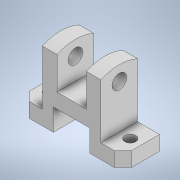
# Autodesk Inventor part: AnchorBase
Saved by Autodesk Inventor 2022.2 (Build 262287030, 287C)
## iProperties
Created: 2023-03-24
Part Number: AnchorBase
Material: Generic
Document SubType Name: Modeling
Designer: jak27277
Mass: 66.295 g
Surface Area: 179.577 cm^2
Volume: 66.295 cm^3
Density: 1 g/cm^3
Appearance: Default
Author: jak27277
Autodesk Inventor part; units mm, degrees
ref_plane "YZ Plane" through (0, 0, 0) normal (1, 0, 0) x (0, 1, 0)
ref_plane "XZ Plane" through (0, 0, 0) normal (0, 1, 0) x (-1, 0, 0)
ref_plane "XY Plane" through (0, 0, 0) normal (0, 0, 1) x (1, 0, 0)
sketch "Sketch2" plane through (0, 0, 0) normal (1, 0, 0) x (0, 1, 0)
  line L0 (-23.6676, 15.875) -> (23.6676, 15.875)
  line L1 (23.6676, 15.875) -> (23.6676, -15.875) construction
  line L2 (23.6676, -15.875) -> (-23.6676, -15.875)
  line L3 (-23.6676, -15.875) -> (-23.6676, 15.875)
  line L4 (-23.6676, 15.875) -> (23.6676, -15.875) construction
  line L5 (23.6676, 15.875) -> (-23.6676, -15.875) construction
  arc A0 (23.6676, -15.875) -> (23.6676, 15.875) centre (-10.9676, 0) ccw
  line L6 (0, 0) -> (-23.6676, 0) construction
  line L7 (27.1324, 0) -> (27.1324, -36.861) construction
  line L8 (-23.6676, 15.875) -> (-36.3676, 15.875)
  line L9 (-36.3676, 15.875) -> (-36.3676, -15.875)
  line L10 (-36.3676, -15.875) -> (-23.6676, -15.875)
  line L11 (-23.6676, -15.875) -> (-23.6676, 15.875)
  dimension "d2" = 38.1
  dimension "d4" = 31.75
  dimension "d5" = 50.8
  dimension "d6" = 12.7
  constraints: 24 end point, 4 parallel, 3 midpoint, 3 point on circle, 2 horizontal, 2 perpendicular, 1 centre point, 1 tangent, 1 vertical, 1 other
  measures "d2" radius of A0
  measures "d4" distance of L2.end L0.start
  measures "d5" distance between parallel lines of L3 L7
  measures "d6" distance of L9.end L10.end
extrude "Extrusion1" add sketch "Sketch2" along normal blind 88.9
sketch "Sketch3" plane through (0, -36.3676, 15.875) normal (0, 0, 1) x (1, 0, 0)
  line L0 (0, 63.5) -> (88.9, 63.5) construction
  line L1 (44.45, 63.5) -> (44.45, 0) construction
  line L2 (0, 0) -> (88.9, 0) construction
  line L3 (31.75, 31.75) -> (57.15, 31.75)
  line L4 (57.15, 31.75) -> (57.15, 63.5)
  line L5 (57.15, 63.5) -> (31.75, 63.5)
  line L6 (31.75, 63.5) -> (31.75, 31.75)
  line L7 (31.75, 31.75) -> (57.15, 63.5) construction
  line L8 (57.15, 31.75) -> (31.75, 63.5) construction
  line L9 (28.575, 19.05) -> (60.325, 19.05)
  line L10 (60.325, 19.05) -> (60.325, 0)
  line L11 (60.325, 0) -> (28.575, 0)
  line L12 (28.575, 0) -> (28.575, 19.05)
  line L13 (28.575, 19.05) -> (60.325, 0) construction
  line L14 (60.325, 19.05) -> (28.575, 0) construction
  line L15 (0, 60.0352) -> (0, 63.5) projected
  line L16 (0, 63.5) -> (19.05, 63.5)
  line L17 (19.05, 63.5) -> (19.05, 12.7)
  line L18 (19.05, 12.7) -> (0, 12.7)
  line L19 (0, 12.7) -> (0, 63.5)
  line L20 (88.9, 63.5) -> (69.85, 63.5)
  line L21 (69.85, 63.5) -> (69.85, 12.7)
  line L22 (69.85, 12.7) -> (88.9, 12.7)
  line L23 (88.9, 12.7) -> (88.9, 63.5)
  point P0 (0, 36.3676)
  point P1 (44.45, 47.625)
  point P2 (44.45, 9.525)
  dimension "d9" = 19.05
  dimension "d10" = 25.4
  dimension "d11" = 31.75
  dimension "d12" = 19.05
  dimension "d13" = 12.7
  dimension "d14" = 50.8
  constraints: 42 end point, 8 parallel, 6 midpoint, 4 horizontal, 4 perpendicular, 4 point on line, 2 equal length
  measures "d9" distance of L21.end L22.end
  measures "d10" distance of L3.start L3.end
  measures "d11" distance of L9.start L9.end
  measures "d12" distance of L9.end L10.end
  measures "d13" distance between parallel lines of L9 L3
  measures "d14" distance of L18.end L0.start
extrude "Extrusion2" cut sketch "Sketch3" against normal through all
sketch "Sketch4" plane through (69.85, -23.6676, 15.875) normal (1, 0, 0) x (0, 0, -1)
  circle A0 centre (15.875, 38.1) radius 6.35
  line L0 (31.75, 0) -> (0, 0) projected
  point P0 (15.875, 23.6676)
  dimension "d17" = 38.1
  dimension "d18" = 12.7
  constraints: 1 centre point, 1 vertical alignment
  measures "d17" distance from line of A0.centre L0
  measures "d18" diameter of A0
extrude "Extrusion3" cut sketch "Sketch4" against normal through all
sketch "Sketch5" plane through (0, -23.6676, 15.875) normal (0, 1, 0) x (1, 0, 0)
  circle A0 centre (9.525, 15.875) radius 4.7625
  circle A1 centre (79.375, 15.875) radius 4.7625
  line L0 (88.9, 31.75) -> (88.9, 0) projected
  line L1 (0, 0) -> (0, 31.75) projected
  line L2 (19.05, 0) -> (0, 0) projected
  line L3 (31.75, 31.75) -> (57.15, 31.75) construction
  line L4 (44.45, 31.75) -> (44.45, 0) construction
  line L5 (57.15, 0) -> (31.75, 0) construction
  line L6 (0, 7.62) -> (7.62, 0)
  line L7 (88.9, 7.62) -> (81.28, 0)
  line L8 (88.9, 0) -> (88.9, 31.75) projected
  line L9 (88.9, 7.62) -> (88.9, 0)
  line L10 (88.9, 0) -> (81.28, 0)
  line L11 (0, 7.62) -> (0, 0)
  line L12 (0, 0) -> (7.62, 0)
  point P0 (0, 15.875)
  dimension "d21" = 9.525
  dimension "d22" = 9.525
  dimension "d24" = 15.875
  dimension "d25" = 7.62
  dimension "d26" = 7.62
  constraints: 14 end point, 2 centre point, 2 collinear, 2 midpoint, 2 point on line, 2 symmetric about line, 1 equal radius, 1 horizontal alignment, 1 perpendicular, 1 other
  measures "d21" diameter of A1
  measures "d22" distance from line of A1.centre L0
  measures "d24" distance from line of L2 A0.centre
  measures "d25" horizontal distance of L6.start L6.end
  measures "d26" horizontal distance of L6.start L6.end
extrude "Extrusion4" cut sketch "Sketch5" against normal through all
body "Solid1"
